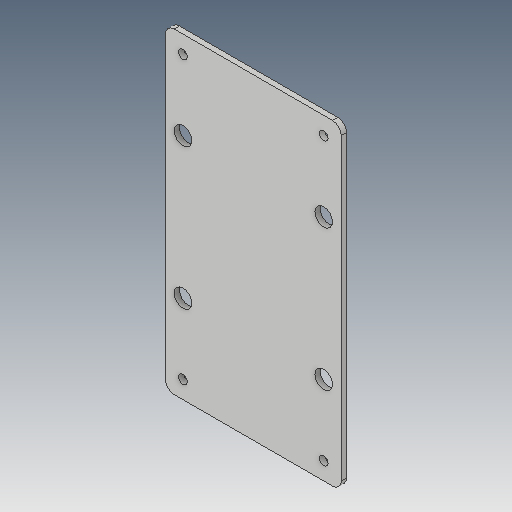
# Autodesk Inventor part: LRFマウント
Saved by Autodesk Inventor 2020.3 (Build 243373000, 373)
## iProperties
Part Number: LRFマウント
Material: 一般
Document SubType Name: Modeling
Designer: highs
Density: 1 g/cm^3
Appearance: 既定
Description: 自作or発注
Stock Number: "自由輪治具 t=3mm d=180mm w=100mm"
Author: highs
Revision Number: カーボン板にする？
Autodesk Inventor part; units mm, degrees
ref_plane "YZ Plane" through (0, 0, 0) normal (1, 0, 0) x (0, 1, 0)
ref_plane "XZ Plane" through (0, 0, 0) normal (0, 1, 0) x (-1, 0, 0)
ref_plane "XY Plane" through (0, 0, 0) normal (0, 0, 1) x (1, 0, 0)
sketch "スケッチ1" plane through (0, 0, 0) normal (0, 0, 1) x (1, 0, 0)
  line L0 (0, 0) -> (100, 0)
  line L1 (100, 0) -> (100, 180)
  line L2 (100, 180) -> (0, 180)
  line L3 (0, 180) -> (0, 0)
  line L4 (0, 10) -> (100, 10) construction
  circle A0 centre (10, 10) radius 2.5
  circle A1 centre (90, 10) radius 2.5
  circle A2 centre (10, 130) radius 5
  circle A3 centre (10, 50) radius 5
  circle A4 centre (90, 130) radius 5
  circle A5 centre (90, 50) radius 5
  line L5 (10, 130) -> (10, 50) construction
  line L6 (10, 50) -> (90, 50) construction
  line L7 (90, 50) -> (90, 130) construction
  line L8 (90, 130) -> (10, 130) construction
  line L9 (0, 90) -> (100, 90) construction
  circle A6 centre (10, 170) radius 2.5
  circle A7 centre (90, 170) radius 2.5
  dimension "d0" = 5
  dimension "d1" = 10
  dimension "d2" = 10
  dimension "d3" = 10
  dimension "d4" = 100
  dimension "d5" = 180
  dimension "d12" = 10
  dimension "d13" = 10
  dimension "d15" = 10
  dimension "d21" = 80
  dimension "d23" = 50
  constraints: 20 end point, 8 centre point, 4 equal radius, 4 perpendicular, 4 point on line, 2 midpoint, 2 parallel, 2 symmetric about line, 1 horizontal, 2 other
  measures "d0" diameter of A0
  measures "d1" distance from line of L3 A0.centre
  measures "d2" distance between parallel lines of L0 L4
  measures "d3" distance from line of L1 A1.centre
  measures "d4" distance of L0.start L0.end
  measures "d5" distance of L2.end L0.start
  measures "d12" diameter of A2
  measures "d13" distance from line of L3 L5.start
  measures "d15" distance from line of L1 L7.end
  measures "d21" distance between parallel lines of L6 L8
  measures "d23" distance between parallel lines of L0 L6
extrude "押し出し1" add sketch "スケッチ1" along normal blind 3
fillet "フィレット1" radius 5 4 edges at (100, 180, 1.5) (0, 180, 1.5) (100, 0, 1.5) (0, 0, 1.5)
